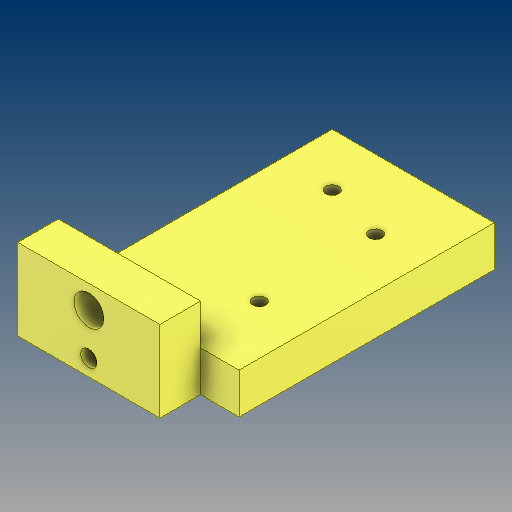
# Autodesk Inventor part: uchwyt_strzykawka_dol
Saved by Autodesk Inventor 2021 (Build 250183000, 183)
## iProperties
Created: 2022-05-15
Part Number: uchwyt_strzykawka_dol
Material: PC/ABS Plastic
Document SubType Name: Modeling
Designer: agnpi
Density: 0.357273 g/cm^3
Appearance: Smooth - Yellow
Author: agnpi
Autodesk Inventor part; units mm, degrees
ref_plane "YZ Plane" through (0, 0, 0) normal (1, 0, 0) x (0, 1, 0)
ref_plane "XZ Plane" through (0, 0, 0) normal (0, 1, 0) x (-1, 0, 0)
ref_plane "XY Plane" through (0, 0, 0) normal (0, 0, 1) x (1, 0, 0)
sketch "Sketch2" plane through (0, 0, 0) normal (0, 1, 0) x (-1, 0, 0)
  line L0 (0, -46.1) -> (0, 56.1) projected
  line L1 (33.556, 0) -> (-28.926, 0) projected
  line L2 (20, -31.5) -> (-20, -31.5)
  line L3 (-20, -31.5) -> (-20, 31.5)
  line L4 (-20, 31.5) -> (20, 31.5)
  line L5 (20, 31.5) -> (20, -31.5)
  line L6 (20, -31.5) -> (-20, 31.5) construction
  line L7 (-20, -31.5) -> (20, 31.5) construction
  line L8 (24.63, 31.5) -> (-10.47, 31.5)
  line L9 (-10.47, 31.5) -> (-10.47, 41.5)
  line L10 (-10.47, 41.5) -> (24.63, 41.5)
  line L11 (24.63, 41.5) -> (24.63, 31.5)
  line L12 (24.63, 31.5) -> (-10.47, 41.5) construction
  line L13 (-10.47, 31.5) -> (24.63, 41.5) construction
  point P0 (0, 0)
  point P1 (7.08, 36.5)
  point P2 (-10.47, 31.5)
  dimension "d5" = 40
  dimension "d6" = 63
  dimension "d7" = 9.53
  dimension "d8" = 35.1
  dimension "d9" = 73
  constraints: 24 end point, 4 midpoint, 4 parallel, 2 horizontal, 2 perpendicular, 1 point on line
  measures "d5" distance of L3.end L4.end
  measures "d6" distance of L2.end L3.end
  measures "d7" distance between parallel lines of L3 L9
  measures "d8" distance between parallel lines of L9 L11
  measures "d9" distance between parallel lines of L2 L10
extrude "Extrusion1" add sketch "Sketch2" along normal blind 10 contours L2 L3 L1 L0 | L0 L1 L5 L2 | L1 L3 L4 L0 | L0 L4 L5 L1
extrude "Extrusion2" add sketch "Sketch2" along normal blind 20 contours L4 L9 L10 L0 | L0 L10 L11 L8 L4
sketch "Sketch3" plane through (0, 10, 0) normal (0, 1, 0) x (1, 0, 0)
  line L0 (-20, 31.5) -> (-20, -31.5) projected
  line L1 (20, 31.5) -> (-20, 31.5) projected
  line L2 (20, -31.5) -> (20, 31.5) projected
  point P0 (0, 0)
  point P1 (-7, 18.5)
  point P2 (-7, -23.5)
  point P3 (7.8, 14.41)
  point P4 (7.8, -14.3)
  dimension "d21" = 13
  dimension "d22" = 13
  dimension "d23" = 42
  dimension "d24" = 13
  dimension "d25" = 12.2
  dimension "d26" = 12.2
  dimension "d27" = 17.09
  dimension "d28" = 28.71
  measures "d21" distance from line of L0 point (-7, 18.5)
  measures "d22" distance from line of L1 point (-7, 18.5)
  measures "d23" distance of point (-7, -23.5) point (-7, 18.5)
  measures "d24" distance from line of L0 point (-7, -23.5)
  measures "d25" distance from line of L2 point (7.8, 14.41)
  measures "d26" distance from line of L2 point (7.8, -14.3)
  measures "d27" distance from line of L1 point (7.8, 14.41)
  measures "d28" distance of point (7.8, -14.3) point (7.8, 14.41)
hole "Hole1" at (-7, 10, -18.5) at (-7, 10, 23.5) at (7.8, 10, -14.41) at (7.8, 10, 14.3) direction (0, -1, 0) diameter 3.242 end through all thread size "M4x0.7" class "6H" standard "ISO Metric profile"
sketch "Sketch4" plane through (-24.63, 0, 41.5) normal (0, 0, 1) x (1, 0, 0)
  line L0 (0, 20) -> (35.1, 20) projected
  line L1 (35.1, 0) -> (35.1, 20) projected
  point P0 (24.63, 0)
  point P1 (17.55, 14.3)
  dimension "d36" = 5.7
  dimension "d37" = 17.55
  measures "d36" distance from line of L0 point (17.55, 14.3)
  measures "d37" distance from line of L1 point (17.55, 14.3)
hole "Hole2" at (-7.08, 14.3, 41.5) direction (0, 0, -1) diameter 7.4 depth 7
sketch "Sketch5" plane through (-24.63, 0, 41.5) normal (0, 0, 1) x (1, 0, 0)
  circle A0 centre (17.55, 14.3) radius 3.7 projected
  line L0 (0, 0) -> (35.1, 0) projected
  line L1 (35.1, 0) -> (35.1, 20) projected
  point P0 (24.63, 0)
  point P1 (17.55, 4)
  dimension "d46" = 4
  dimension "d47" = 17.55
  measures "d46" distance from line of L0 point (17.55, 4)
  measures "d47" distance from line of L1 point (17.55, 4)
hole "Hole3" at (-7.08, 4, 41.5) direction (0, 0, -1) diameter 4 depth 7
body "Solid1"
